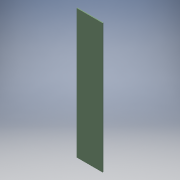
# Autodesk Inventor part: Foil
Saved by Autodesk Inventor 2019 (Build 230136000, 136)
## iProperties
Created: 2017-01-18
Part Number: Foil
Document SubType Name: Modeling
Designer: Administrator
Density: 1 g/cm^3
Mass: 0.036 g
Surface Area: 3.744 cm^2
Volume: 0.036 cm^3
Material: Generic
Appearance: Green Pastel
Author: Administrator
Autodesk Inventor part; units mm, degrees
ref_plane "YZ Plane" through (0, 0, 0) normal (1, 0, 0) x (0, 1, 0)
ref_plane "XZ Plane" through (0, 0, 0) normal (0, 1, 0) x (-1, 0, 0)
ref_plane "XY Plane" through (0, 0, 0) normal (0, 0, 1) x (1, 0, 0)
sketch "Sketch1" plane through (0, 0, 0) normal (0, 0, 1) x (1, 0, 0)
  line L0 (0, 0) -> (6, 0)
  line L1 (6, 0) -> (6, 0.2)
  line L2 (6, 0.2) -> (0, 0.2)
  line L3 (0, 0.2) -> (0, 0)
  dimension "d0" = 0.2
  dimension "d1" = 6
  constraints: 8 end point, 2 parallel, 1 horizontal, 1 perpendicular, 1 other
  measures "d0" distance of L0.end L1.end
  measures "d1" distance of L0.start L0.end
extrude "Extrusion1" add sketch "Sketch1" along normal blind 30
body "Solid1"
